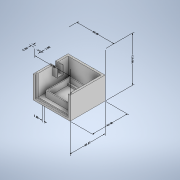
# Autodesk Inventor part: Part_C1
Saved by Autodesk Inventor 2022.6 (Build 266554010, 554A)
## iProperties
Created: 2025-05-16
Part Number: Part_C1
Material: Generic
Document SubType Name: Modeling
Designer: khinm
Density: 1 g/cm^3
Appearance: Default
Author: khinm
Autodesk Inventor part; units mm, degrees
ref_plane "YZ Plane" through (0, 0, 0) normal (1, 0, 0) x (0, 1, 0)
ref_plane "XZ Plane" through (0, 0, 0) normal (0, 1, 0) x (-1, 0, 0)
ref_plane "XY Plane" through (0, 0, 0) normal (0, 0, 1) x (1, 0, 0)
sketch "Sketch1" plane through (0, 0, 0) normal (0, 0, 1) x (1, 0, 0)
  line L0 (-45, 55) -> (45, 55)
  line L1 (45, 55) -> (45, -55)
  line L2 (45, -55) -> (-45, -55)
  line L3 (-45, -55) -> (-45, 55)
  point P0 (0, 0)
  point P1 (0, 55)
  point P2 (-45, 0)
  dimension "d0" = 110
  dimension "d1" = 90
  constraints: 8 end point, 2 midpoint, 2 parallel, 1 horizontal, 1 horizontal alignment, 1 perpendicular, 1 vertical alignment
  measures "d0" distance between parallel lines of L2 L0
  measures "d1" distance of L1.end L2.end
extrude "Extrusion1" add sketch "Sketch1" along normal mid plane 85
sketch "Sketch2" plane through (0, 0, 42.5) normal (0, 0, 1) x (1, 0, 0)
  line L0 (-40, 50) -> (40, 50)
  line L1 (40, 50) -> (40, -50)
  line L2 (40, -50) -> (-40, -50)
  line L3 (-40, -50) -> (-40, 50)
  line L4 (45, 55) -> (-45, 55) projected
  line L5 (-45, 55) -> (-45, -55) projected
  point P0 (0, 0)
  point P1 (0, 50)
  point P2 (0, -50)
  point P3 (-40, 0)
  point P4 (40, 0)
  dimension "d6" = 5
  dimension "d7" = 5
  constraints: 8 end point, 4 midpoint, 2 horizontal alignment, 2 parallel, 2 vertical alignment, 1 horizontal, 1 perpendicular
  measures "d6" distance between parallel lines of L0 L4
  measures "d7" distance between parallel lines of L5 L3
extrude "Extrusion2" cut sketch "Sketch2" against normal blind 80
sketch "Sketch3" plane through (-45, 55, 42.5) normal (0, 1, 0) x (1, 0, 0)
  line L0 (2, 7) -> (88, 7)
  line L1 (88, 7) -> (88, 2)
  line L2 (2, 2) -> (2, 7)
  line L3 (90, 0) -> (0, 0) projected
  line L4 (0, 85) -> (0, 0) projected
  line L5 (7, 2) -> (7, 0)
  line L6 (85, 0) -> (5, 0) projected
  line L7 (83, 2) -> (83, 0)
  line L8 (88, 2) -> (83, 2)
  line L9 (7, 2) -> (2, 2)
  line L10 (7, 0) -> (83, 0)
  point P0 (45, 42.5)
  point P1 (45, 7)
  point P2 (2, 4.5)
  point P3 (7, 0)
  dimension "d14" = 2
  dimension "d15" = 5
  dimension "d16" = 7
  dimension "d17" = 7
  dimension "d18" = 7
  dimension "d19" = 5
  constraints: 16 end point, 3 parallel, 3 perpendicular, 2 midpoint, 2 point on line, 1 collinear, 1 horizontal, 1 vertical alignment
  measures "d14" distance from line of L4 point (2, 4.5)
  measures "d15" distance of L1.end L0.end
  measures "d16" distance of L3.end L5.end
  measures "d17" distance of L3.start L7.end
  measures "d18" distance between parallel lines of L3 L0
  measures "d19" distance between parallel lines of L9 L0
extrude "Extrusion3" cut sketch "Sketch3" against normal up to surface (105 mm away)
sketch "Sketch4" plane through (-40, -50, 42.5) normal (0, 1, 0) x (1, 0, 0)
  line L0 (-3, 7) -> (83, 7)
  line L1 (83, 7) -> (83, 2)
  line L2 (83, 2) -> (-3, 2)
  line L3 (-3, 2) -> (-3, 7)
  line L4 (80, 0) -> (0, 0) projected
  point P0 (40, 42.5)
  point P1 (40, 2)
  point P2 (40, 0)
  point P3 (83, 4.5)
  point P4 (-3, 4.5)
  dimension "d22" = 2
  dimension "d23" = 86
  dimension "d24" = 5
  constraints: 8 end point, 4 midpoint, 2 parallel, 1 horizontal, 1 perpendicular, 1 vertical alignment
  measures "d22" distance between parallel lines of L4 L2
  measures "d23" distance of point (83, 4.5) point (-3, 4.5)
  measures "d24" distance of L1.end L0.end
extrude "Extrusion4" cut sketch "Sketch4" against normal blind 3
sketch "Sketch5" plane through (-40, -50, -37.5) normal (0, 1, 0) x (1, 0, 0)
  line L0 (80, 0) -> (0, 0) projected
  line L1 (11.85, -8) -> (68.15, -8)
  line L2 (68.15, -8) -> (68.15, -62.2)
  line L3 (68.15, -62.2) -> (11.85, -62.2)
  line L4 (11.85, -62.2) -> (11.85, -8)
  point P0 (40, -37.5)
  point P1 (40, -8)
  dimension "d37" = 56.3
  dimension "d38" = 54.2
  dimension "d39" = 8
  constraints: 8 end point, 2 parallel, 1 horizontal, 1 midpoint, 1 perpendicular, 1 vertical alignment
  measures "d37" distance of L1.start L1.end
  measures "d38" distance of L1.end L2.end
  measures "d39" distance between parallel lines of L1 L0
sketch "Sketch6" plane through (-40, -50, -37.5) normal (0, 1, 0) x (1, 0, 0)
  line L0 (9.85, -6) -> (70.15, -6)
  line L1 (70.15, -6) -> (70.15, -64.2)
  line L2 (70.15, -64.2) -> (9.85, -64.2)
  line L3 (9.85, -64.2) -> (9.85, -6)
  line L4 (80, 0) -> (0, 0) projected
  point P0 (40, -37.5)
  point P1 (40, -6)
  dimension "d40" = 58.2
  dimension "d41" = 60.3
  dimension "d42" = 6
  constraints: 8 end point, 2 parallel, 1 horizontal, 1 midpoint, 1 perpendicular, 1 vertical alignment
  measures "d40" distance of L0.end L1.end
  measures "d41" distance of L0.start L0.end
  measures "d42" distance between parallel lines of L4 L0
extrude "Extrusion5" add sketch "Sketch6" along normal blind 15
extrude "Extrusion6" cut sketch "Sketch5" along normal up to surface (15 mm away)
sketch "Sketch8" plane through (-40, -50, -37.5) normal (0, 1, 0) x (1, 0, 0)
  line L0 (11.85, -8) -> (68.15, -8) projected
  line L1 (68.15, -8) -> (68.15, -62.2) projected
  line L2 (11.85, -8) -> (68.15, -8)
  line L3 (68.15, -8) -> (68.15, -13)
  line L4 (68.15, -13) -> (11.85, -13)
  line L5 (11.85, -13) -> (11.85, -8)
  point P0 (40, -37.5)
  dimension "d48" = 5
  constraints: 8 end point, 2 parallel, 1 horizontal, 1 perpendicular, 1 point on line
  measures "d48" distance between parallel lines of L0 L4
extrude "Extrusion7" add sketch "Sketch8" along normal blind 4
sketch "Sketch10" plane through (-40, -50, -37.5) normal (1, 0, 0) x (0, 0, -1)
  line L0 (-25.5, 83) -> (-36.5, 83)
  line L1 (-36.5, 83) -> (-36.5, 29.5)
  line L2 (-36.5, 29.5) -> (-25.5, 29.5)
  line L3 (-25.5, 29.5) -> (-25.5, 83)
  line L4 (-8, 4) -> (-8, 15) projected
  line L5 (0, 0) -> (0, 100) projected
  line L6 (-13, 0) -> (-62.2, 0) projected
  point P0 (-37.5, 50)
  dimension "d52" = 25.5
  dimension "d53" = 11
  dimension "d54" = 29.5
  dimension "d55" = 53.5
  constraints: 8 end point, 2 parallel, 1 horizontal, 1 perpendicular
  measures "d52" distance between parallel lines of L3 L5
  measures "d53" distance between parallel lines of L3 L1
  measures "d54" distance between parallel lines of L6 L2
  measures "d55" distance of L2.end L0.start
extrude "Extrusion8" cut sketch "Sketch10" against normal up to surface (5 mm away)
sketch "Sketch11" plane through (-40, -50, -37.5) normal (1, 0, 0) x (0, 0, -1)
  line L0 (-38, 84.5) -> (-24, 84.5)
  line L1 (-24, 84.5) -> (-24, 28)
  line L2 (-24, 28) -> (-38, 28)
  line L3 (-38, 28) -> (-38, 84.5)
  line L4 (-36.5, 83) -> (-25.5, 83) projected
  line L5 (-36.5, 29.5) -> (-36.5, 83) projected
  point P0 (-37.5, 50)
  point P1 (-31, 84.5)
  point P2 (-31, 83)
  point P3 (-38, 56.25)
  point P4 (-36.5, 56.25)
  dimension "d58" = 1.5
  dimension "d59" = 1.5
  constraints: 8 end point, 4 midpoint, 2 parallel, 1 horizontal, 1 horizontal alignment, 1 perpendicular, 1 vertical alignment
  measures "d58" distance between parallel lines of L3 L5
  measures "d59" distance from line of L4.end L0
extrude "Extrusion9" add sketch "Sketch11" along normal up to surface (11.85 mm away)
sketch "Sketch12" plane through (-28.15, -22, 0.5) normal (1, 0, 0) x (0, 0, -1)
  line L0 (12.5, 1.5) -> (12.5, 55) projected
  line L1 (1.5, 55) -> (12.5, 55)
  line L2 (12.5, 55) -> (12.5, 1.5)
  line L3 (12.5, 1.5) -> (1.5, 1.5)
  line L4 (1.5, 1.5) -> (1.5, 55)
  line L5 (14, 56.5) -> (0, 56.5) projected
  line L6 (0, 56.5) -> (0, 0) projected
  point P0 (0.5, 22)
  point P1 (7, 55)
  point P2 (7, 56.5)
  point P3 (0, 28.25)
  point P4 (1.5, 28.25)
  dimension "d62" = 1.5
  constraints: 8 end point, 4 midpoint, 2 parallel, 1 horizontal, 1 horizontal alignment, 1 perpendicular, 1 point on line, 1 vertical alignment
  measures "d62" distance between parallel lines of L5 L1
extrude "Extrusion10" cut sketch "Sketch12" against normal up to surface (11.85 mm away)
body "Solid1"
